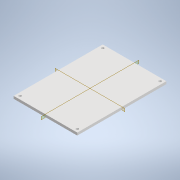
# Autodesk Inventor part: A-00
Saved by Autodesk Inventor 2022.2 (Build 262287000, 287)
## iProperties
Created: 2021-12-01
Part Number: A-00
Material: Generic
Document SubType Name: Modeling
Designer: kfcs7
Density: 1 g/cm^3
Appearance: Default
Author: kfcs7
Autodesk Inventor part; units mm, degrees
ref_plane "YZ Plane" through (0, 0, 0) normal (1, 0, 0) x (0, 1, 0)
ref_plane "XZ Plane" through (0, 0, 0) normal (0, 1, 0) x (-1, 0, 0)
ref_plane "XY Plane" through (0, 0, 0) normal (0, 0, 1) x (1, 0, 0)
sketch "Sketch1" plane through (0, 0, 0) normal (0, 1, 0) x (-1, 0, 0)
  line L0 (25, 35) -> (-25, 35)
  line L1 (-25, 35) -> (-25, -35)
  line L2 (-25, -35) -> (25, -35)
  line L3 (25, -35) -> (25, 35)
  line L4 (25, 35) -> (-25, -35) construction
  line L5 (-25, 35) -> (25, -35) construction
  point P0 (0, 0)
  dimension "d0" = 50
  dimension "d1" = 70
  constraints: 12 end point, 2 midpoint, 2 parallel, 1 horizontal, 1 perpendicular
  measures "d0" distance of L2.end L1.end
  measures "d1" distance of L1.end L0.end
extrude "Extrusion1" add sketch "Sketch1" along normal blind 2
sketch "Sketch2" plane through (0, 2, 0) normal (0, 1, 0) x (1, 0, 0)
  line L0 (-22.5, -32.5) -> (22.5, -32.5) construction
  line L1 (22.5, -32.5) -> (22.5, 32.5) construction
  line L2 (22.5, 32.5) -> (-22.5, 32.5) construction
  line L3 (-22.5, 32.5) -> (-22.5, -32.5) construction
  line L4 (-22.5, -32.5) -> (22.5, 32.5) construction
  line L5 (22.5, -32.5) -> (-22.5, 32.5) construction
  circle A0 centre (-22.5, 32.5) radius 1
  circle A1 centre (-22.5, -32.5) radius 1
  circle A2 centre (22.5, -32.5) radius 1
  circle A3 centre (22.5, 32.5) radius 1
  point P0 (0, 0)
  dimension "d4" = 45
  dimension "d5" = 65
  dimension "d6" = 2
  constraints: 12 end point, 4 centre point, 3 coincident, 3 equal radius, 2 midpoint, 2 parallel, 1 horizontal, 1 perpendicular
  measures "d4" distance of L2.end L1.end
  measures "d5" distance of L1.end L0.end
  measures "d6" diameter of A0
extrude "Extrusion2" cut sketch "Sketch2" against normal through all
ref_plane "Work Plane1" through (0, 0, -35) normal (-1, 0, 0) x (0, 0, 1)
ref_plane "Work Plane2" through (-25, 0, 0) normal (0, 0, 1) x (1, 0, 0)
body "Solid1"
